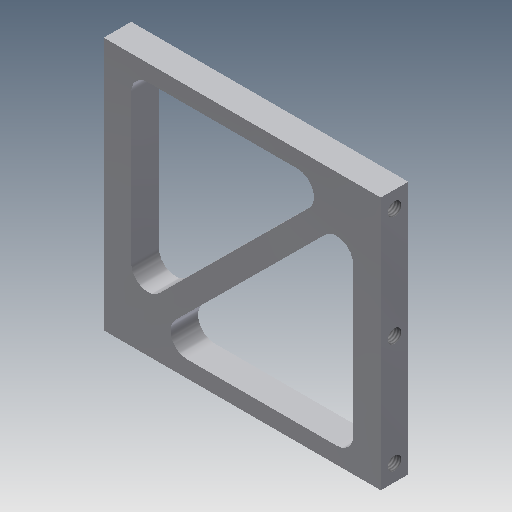
# Autodesk Inventor part: リンク_ふともも_サブフレーム_1_1(予備案)
Saved by Autodesk Inventor 2017.3 (Build 213256000, 256)
## iProperties
Created: 2016-06-02
Part Number: リンク_ふともも_サブフレーム_1_1(予備案)
Material: アルミニウム 2014-T4
Document SubType Name: Modeling
Designer: hiroaki
Density: 2.8 g/cm^3
Appearance: サテン
Author: hiroaki
Autodesk Inventor part; units mm, degrees
ref_plane "YZ Plane" through (0, 0, 0) normal (1, 0, 0) x (0, 1, 0)
ref_plane "XZ Plane" through (0, 0, 0) normal (0, 1, 0) x (-1, 0, 0)
ref_plane "XY Plane" through (0, 0, 0) normal (0, 0, 1) x (1, 0, 0)
sketch "スケッチ1" plane through (0, 0, 0) normal (0, 0, 1) x (1, 0, 0)
  line L0 (-25.15, -23) -> (25.15, -23)
  line L1 (25.15, -23) -> (25.15, 23)
  line L2 (25.15, 23) -> (-25.15, 23)
  line L3 (-25.15, 23) -> (-25.15, -23)
  line L4 (-25.15, -23) -> (25.15, 23) construction
  line L5 (25.15, -23) -> (-25.15, 23) construction
  line L6 (-25.15, 20) -> (25.15, 20) construction
  line L7 (-25.15, -20) -> (25.15, -20) construction
  line L8 (-25.15, 20) -> (-25.15, -20) construction
  line L9 (-20.15, 20) -> (-20.15, -17.1821)
  line L10 (-20.15, -17.1821) -> (17.3109, 20)
  line L11 (17.3109, 20) -> (-20.15, 20)
  line L12 (-20.15, -20) -> (20.15, -20) construction
  line L13 (20.15, -20) -> (20.15, 20) construction
  line L14 (20.15, 20) -> (-20.15, 20) construction
  line L15 (-20.15, 20) -> (-20.15, -20) construction
  line L16 (-20.15, -20) -> (20.15, 20) construction
  line L17 (20.15, -20) -> (-20.15, 20) construction
  line L18 (20.15, 17.1821) -> (20.15, -20)
  line L19 (20.15, -20) -> (-17.3109, -20)
  line L20 (-17.3109, -20) -> (20.15, 17.1821)
  point P0 (0, 0)
  point P1 (-25.15, 0)
  point P2 (0, 0)
  dimension "d1" = 50.3
  dimension "d3" = 40
  dimension "d5" = 3
  dimension "d9" = 5
  dimension "d16" = 3
  dimension "d17" = 2
  constraints: 42 end point, 7 parallel, 6 midpoint, 4 collinear, 4 perpendicular, 4 point on line, 3 vertical, 2 horizontal, 1 horizontal alignment, 1 other
  measures "d1" distance of L1.end L2.end
  measures "d3" distance between parallel lines of L7 L6
  measures "d5" distance between parallel lines of L2 L6
  measures "d9" distance between parallel lines of L8 L15
  measures "d16" distance between parallel lines of L2 L14
  measures "d17" distance between parallel lines of L16 L10
extrude "押し出し1" add sketch "スケッチ1" along normal blind 5
fillet "フィレット1" radius 3 6 edges at (-20.15, -17.1821, 2.5) (-17.3109, -20, 2.5) (-20.15, 20, 2.5) (17.3109, 20, 2.5) (20.15, 17.1821, 2.5) (20.15, -20, 2.5)
sketch "スケッチ2" plane through (25.15, -23, 0) normal (1, 0, 0) x (0, 0, -1)
  line L0 (0, 46) -> (-5, 46) projected
  line L1 (-5, 0) -> (-5, 46) projected
  point P0 (0, 23)
  point P1 (-2.5, 3)
  point P2 (-2.5, 43)
  point P3 (-2.5, 23)
  point P4 (-2.5, 46)
  point P5 (-5, 23)
  dimension "d21" = 40
  dimension "d22" = 20
  constraints: 3 vertical alignment, 2 midpoint, 1 horizontal alignment
  measures "d21" distance of point (-2.5, 43) point (-2.5, 3)
  measures "d22" distance of point (-2.5, 43) point (-2.5, 23)
hole "穴1" at (25.15, -20, 2.5) at (25.15, 20, 2.5) at (25.15, 0, 2.5) direction (-1, 0, 0) diameter 2.459 depth 3 thread size "M3x0.5" class "6H" standard "ISO Metric profile"
mirror "ミラー1" about plane through (0, 0, 0) normal (1, 0, 0) of "穴1"
equation "\"d3\" = d13"
equation "\"d21\" = d3"
equation "\"d22\" = 0.5 * d21"
equation "\"d13\" = 40"
